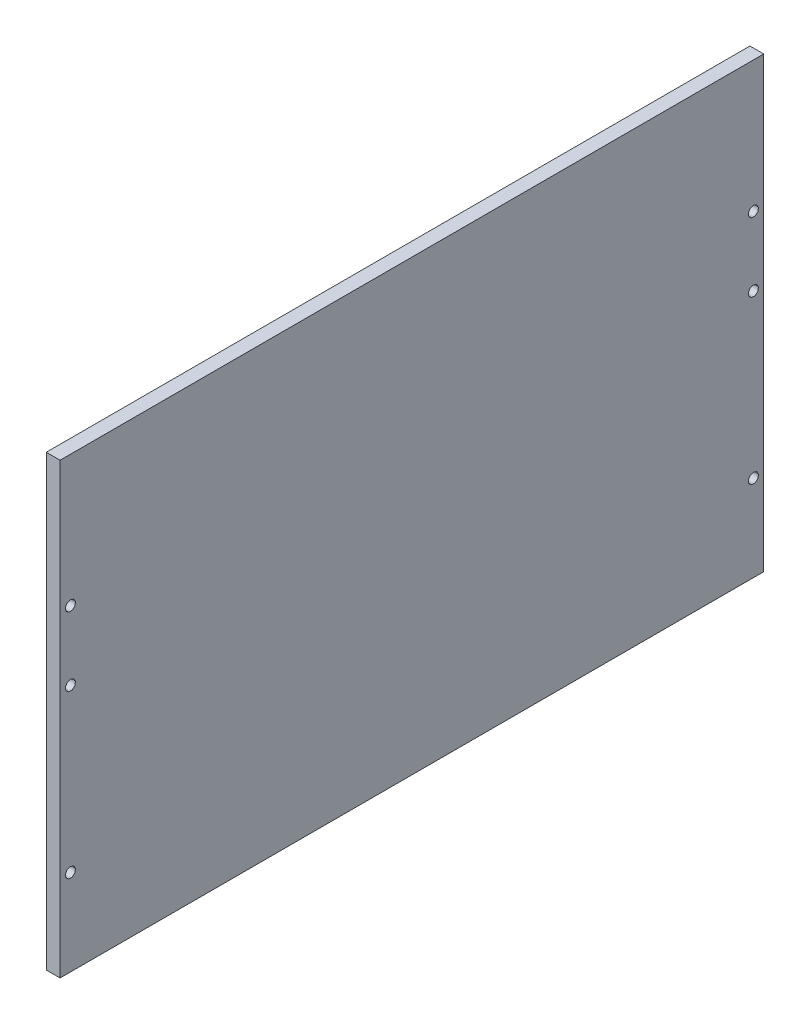
# Autodesk Inventor part: крышка
Saved by Autodesk Inventor 2024.2 (Build 282272000, 272)
## iProperties
Created: 2026-02-12
Part Number: крышка
Material: Типовые
Document SubType Name: Modeling
Designer: Service
Density: 1 g/cm^3
Appearance: По умолчанию
Author: Service
Autodesk Inventor part; units mm, degrees
ref_plane "YZ Plane" through (0, 0, 0) normal (1, 0, 0) x (0, 1, 0)
ref_plane "XZ Plane" through (0, 0, 0) normal (0, 1, 0) x (-1, 0, 0)
ref_plane "XY Plane" through (0, 0, 0) normal (0, 0, 1) x (1, 0, 0)
sketch "Эскиз1" plane through (0, 0, 0) normal (1, 0, 0) x (0, 1, 0)
  line L0 (70.9825, 98.2222) -> (-59.0175, 98.2222)
  line L1 (-59.0175, 98.2222) -> (-59.0175, -105.7778)
  line L2 (-59.0175, -105.7778) -> (70.9825, -105.7778)
  line L3 (70.9825, -105.7778) -> (70.9825, 98.2222)
  circle A0 centre (-34.0175, 95.2222) radius 1.5
  circle A1 centre (-34.0175, -102.7778) radius 1.5
  circle A2 centre (12.9825, 95.2222) radius 1.5
  circle A3 centre (12.9825, -102.7778) radius 1.5
  circle A4 centre (32.9825, 95.2222) radius 1.5
  circle A5 centre (32.9825, -102.7778) radius 1.5
  point P0 (0, 0)
  dimension "d0" = 204
  dimension "d1" = 130
  dimension "d2" = 3
  dimension "d3" = 25
  dimension "d4" = 25
  dimension "d5" = 3
  dimension "d6" = 3
  dimension "d7" = 3
  dimension "d8" = 72
  dimension "d9" = 3
  dimension "d10" = 3
  dimension "d11" = 3
  dimension "d12" = 72
  dimension "d13" = 3
  dimension "d14" = 3
  dimension "d15" = 20
  dimension "d16" = 3
  dimension "d17" = 3
  dimension "d18" = 20
  constraints: 8 end point, 6 centre point, 2 parallel, 1 equal radius, 1 horizontal, 1 perpendicular
  measures "d0" distance of L2.end L0.start
  measures "d1" distance of L0.start L0.end
  measures "d2" diameter of A0
  measures "d3" distance from line of L1 A0.centre
  measures "d4" distance from line of L1 A1.centre
  measures "d5" distance from line of L0 A0.centre
  measures "d6" distance from line of L2 A1.centre
  measures "d7" diameter of A2
  measures "d8" distance from line of A2.centre L1
  measures "d9" distance from line of L0 A2.centre
  measures "d10" diameter of A3
  measures "d11" distance from line of A3.centre L2
  measures "d12" distance from line of L1 A3.centre
  measures "d13" diameter of A4
  measures "d14" distance from line of L0 A4.centre
  measures "d15" distance of A2.centre A4.centre
  measures "d16" diameter of A5
  measures "d17" distance from line of L2 A5.centre
  measures "d18" distance of A3.centre A5.centre
extrude "Выдавливание1" add sketch "Эскиз1" along normal blind 4
